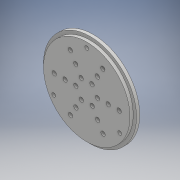
# Autodesk Inventor part: bearing-base-uppercase
Saved by Autodesk Inventor 2018 (Build 220112000, 112)
## iProperties
Created: 2025-02-23
Part Number: bearing-base-uppercase
Material: Generic
Document SubType Name: Modeling
Designer: neo
Density: 1 g/cm^3
Appearance: Default
Author: neo
Autodesk Inventor part; units mm, degrees
ref_plane "YZ Plane" through (0, 0, 0) normal (1, 0, 0) x (0, 1, 0)
ref_plane "XZ Plane" through (0, 0, 0) normal (0, 1, 0) x (-1, 0, 0)
ref_plane "XY Plane" through (0, 0, 0) normal (0, 0, 1) x (1, 0, 0)
sketch "Sketch1" plane through (0, 0, 0) normal (0, 0, 1) x (1, 0, 0)
  line L0 (17.9921, 17.8802) -> (17.9921, -20.5689)
  line L1 (-32.0079, 4.8802) -> (-32.0079, 14.8802) construction
  line L2 (-32.0079, 14.8802) -> (-22.0079, 14.8802) construction
  line L3 (-22.0079, 14.8802) -> (-22.0079, 4.8802) construction
  line L4 (-22.0079, 4.8802) -> (-32.0079, 4.8802) construction
  line L5 (-32.0079, 4.8802) -> (-32.0079, 14.8802) construction
  line L6 (17.9921, 14.8802) -> (-31.6168, 14.8802) construction
  line L7 (-31.6168, 4.8802) -> (18.3832, 4.8802) construction
  line L8 (-22.0079, 14.8802) -> (17.9921, 14.8802)
  line L9 (17.9921, 11.8802) -> (-22.0079, 11.8802)
  line L10 (-22.0079, 11.8802) -> (-22.0079, 14.8802)
  line L11 (17.9921, 14.8802) -> (17.9921, 11.8802)
  line L12 (-25.0079, 14.8802) -> (17.9921, 14.8802)
  line L13 (17.9921, 14.8802) -> (17.9921, 17.8802)
  line L14 (17.9921, 17.8802) -> (-25.0079, 17.8802)
  line L15 (-25.0079, 17.8802) -> (-25.0079, 14.8802)
  point P0 (0, 0)
  dimension "d2" = 10
  dimension "d13" = 10
  dimension "d52" = 3
  dimension "d53" = 0
  dimension "d55" = 80
  dimension "d56" = 40
  dimension "d57" = 3
  dimension "d58" = 3
  constraints: 32 end point, 5 parallel, 3 horizontal, 3 perpendicular, 2 point on line, 1 vertical
  measures "d2" distance between parallel lines of L1 L3
  measures "d13" distance between parallel lines of L7 L6
  measures "d52" distance between parallel lines of L9 L8
  measures "d53" distance between parallel lines of L2 L6
  measures "d55" diameter of L3 L0
  measures "d56" distance between parallel lines of L3 L11
  measures "d57" distance between parallel lines of L6 L14
  measures "d58" distance between parallel lines of L10 L15
revolve "Revolution1" add sketch "Sketch1" angle 360 about axis through (17.9921, 17.8802, 0) along (0, -1, 0)
sketch "Sketch3" plane through (17.9921, 11.8802, 0) normal (0, -1, 0) x (1, 0, 0)
  circle A0 centre (0, 0) radius 40 projected
  line L0 (0, 40) -> (0, -38.6275)
  line L1 (-39.9999, 0.0946) -> (39.9999, 0.0946)
  circle A1 centre (10, 0.0946) radius 2
  circle A2 centre (20, 0.0946) radius 2
  circle A3 centre (30, 0.0946) radius 2
  circle A4 centre (4.9181, 8.7075) radius 2
  circle A5 centre (9.9181, 17.3678) radius 2
  circle A6 centre (14.9181, 26.028) radius 2
  circle A7 centre (-5.0819, 8.613) radius 2
  circle A8 centre (-10.0819, 17.2732) radius 2
  circle A9 centre (-15.0819, 25.9335) radius 2
  circle A10 centre (-10, -0.0946) radius 2
  circle A11 centre (-20, -0.0946) radius 2
  circle A12 centre (-30, -0.0946) radius 2
  circle A13 centre (-4.9181, -8.7075) radius 2
  circle A14 centre (-9.9181, -17.3678) radius 2
  circle A15 centre (-14.9181, -26.028) radius 2
  circle A16 centre (5.0819, -8.613) radius 2
  circle A17 centre (10.0819, -17.2732) radius 2
  circle A18 centre (15.0819, -25.9335) radius 2
  circle A19 centre (0, 35.25) radius 1.75
  circle A20 centre (-30.5274, -17.625) radius 1.75
  circle A21 centre (30.5274, -17.625) radius 1.75
  circle A22 centre (0, 0) radius 37 construction
  point P0 (-17.9921, 0)
  dimension "d59" = 4
  dimension "d60" = 10
  dimension "d66" = 10
  dimension "d70" = 360
  dimension "d72" = 3.5
  dimension "d75" = 360
  dimension "d80" = 3
  constraints: 22 centre point, 4 end point, 3 point on circle, 2 horizontal, 2 point on line, 1 coincident, 1 tangent, 1 vertical, 48 other
  measures "d59" diameter of A1
  measures "d60" horizontal distance of A0.centre A1.centre
  measures "d66" distance of A1.centre A2.centre
  measures "d72" diameter of A19
  measures "d80" radial gap between concentric circles of A22 A0
extrude "Extrusion2" cut sketch "Sketch3" against normal through all contours A3 L1 | L1 A3 | A12 L1 | L1 A12 | A19 L0 | L0 A19 | A2 L1 | L1 A2 | A11 L1 | L1 A11 | A10 L1 | L1 A10 | A1 L1 | L1 A1 | A4 | A5 | A6 | A7 | A8 | A9 | A13 | A14 | A15 | A16 | A17 | A18 | A20 | A21
body "Solid1"
